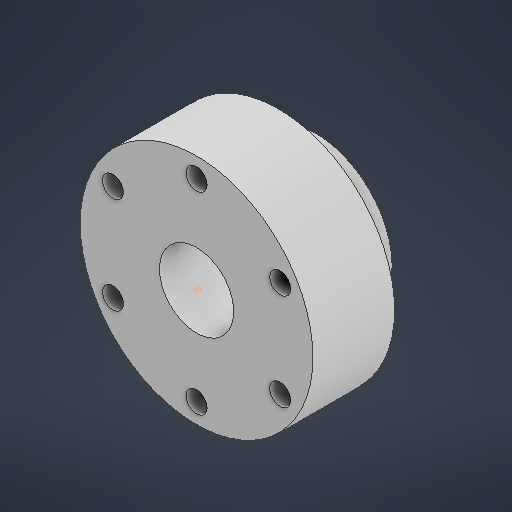
# Autodesk Inventor part: Porsche_912_CV_Joint
Saved by Autodesk Inventor 2026.1 (Build 301233000, 233)
## iProperties
Created: 2026-08-06
Part Number: Porsche_912_CV_Joint
Material: Generic
Document SubType Name: Modeling
Designer: share
Density: 1 g/cm^3
Appearance: Default
Author: share
Autodesk Inventor part; units mm, degrees
ref_plane "YZ Plane" through (0, 0, 0) normal (1, 0, 0) x (0, 1, 0)
ref_plane "XZ Plane" through (0, 0, 0) normal (0, 1, 0) x (-1, 0, 0)
ref_plane "XY Plane" through (0, 0, 0) normal (0, 0, 1) x (1, 0, 0)
sketch "Sketch1" plane through (0, 0, 0) normal (0, 0, 1) x (1, 0, 0)
  circle A0 centre (0, 0) radius 47
  dimension "d24" = 94
  constraints: 1 centre point, 1 coincident
  measures "d24" diameter of A0
extrude "Extrusion1" add sketch "Sketch1" along normal blind 33
sketch "Sketch3" plane through (0, 0, 0) normal (0, 0, 1) x (1, 0, 0)
  circle A0 centre (0, 0) radius 31
  dimension "d21" = 62
  constraints: 1 centre point, 1 coincident
  measures "d21" diameter of A0
extrude "Extrusion2" add sketch "Sketch3" against normal blind 15
sketch "Sketch4" plane through (0, 0, 33) normal (0, 0, 1) x (1, 0, 0)
  circle A0 centre (0, 0) radius 39 construction
  line L0 (0, 0) -> (0, 39) construction
  dimension "d25" = 78
  constraints: 2 coincident, 2 end point, 1 vertical, 1 vertical alignment, 2 other
hole "Hole2" at (0, 39, 33) direction (0, 0, -1) diameter 8.5 end through all
pattern_circular "Circular Pattern2" count 6 over 360 about axis through (0, 0, -10) along (0, 0, 1) of "Hole2"
sketch "Sketch5" plane through (0, 0, 0) normal (0, 0, 1) x (1, 0, 0)
  circle A0 centre (0, 0) radius 15
  dimension "d36" = 30
  constraints: 1 centre point, 1 coincident
  measures "d36" diameter of A0
extrude "Extrusion3" cut sketch "Sketch5" along normal through all both and the other way through all
body "Solid1"
